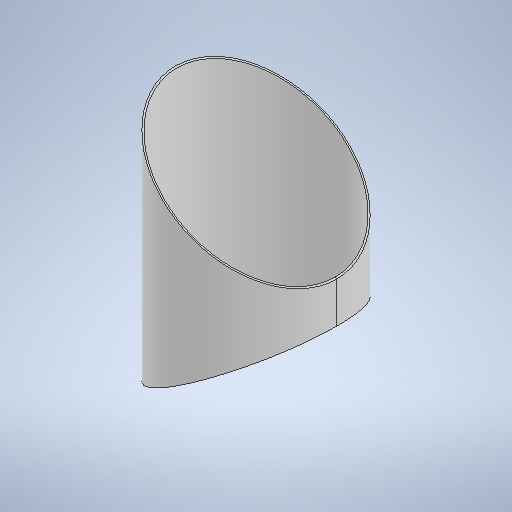
# Autodesk Inventor part: GBK-RK-0032 tube segmeng 2
Saved by Autodesk Inventor 2026.2 (Build 302298000, 298)
## iProperties
Created: 2026-09-14
Part Number: GBK-RK-0032 tube segmeng 2
Material: Generic
Document SubType Name: Sheet Metal
Designer: admin
Density: 1 g/cm^3
Flat Pattern Width: 101.018 cm
Flat Pattern Length: 50 cm
Flat Pattern Area: 5050.91 cm^2
Sheet Metal Rule: Default_mm
Sheet Metal Width: 1010,181 mm
Sheet Metal Length: 500,000 mm
Sheet Metal Area: 505090,589 mm^2
Appearance: Default
Author: admin
Autodesk Inventor part; units mm, degrees
ref_plane "YZ Plane" through (0, 0, 0) normal (1, 0, 0) x (0, 1, 0)
ref_plane "XZ Plane" through (0, 0, 0) normal (0, 1, 0) x (-1, 0, 0)
ref_plane "XY Plane" through (0, 0, 0) normal (0, 0, 1) x (1, 0, 0)
sketch "Sketch1" plane through (0, 0, 0) normal (0, 0, 1) x (1, 0, 0)
  line L0 (0, 0) -> (0, 204.8418)
  line L1 (159.5, 0) -> (162.5, 0)
  line L2 (162.5, 0) -> (162.5, 500)
  line L3 (162.5, 500) -> (159.5, 500)
  line L4 (159.5, 500) -> (159.5, 0)
  dimension "d0" = 3
  dimension "d1" = 500
  dimension "d2" = 325
  constraints: 10 end point, 2 parallel, 1 horizontal, 1 perpendicular, 1 point on line, 1 vertical
  measures "d0" distance of L3.end L2.end
  measures "d1" distance of L2.end L1.end
  measures "d2" diameter of L2 L0
revolve "Revolution1" add sketch "Sketch1" angle 359.9 about axis through (0, 0, 0) along (0, 1, 0)
sketch "Sketch2" plane through (0, 0, 0) normal (0, 0, 1) x (1, 0, 0)
  line L0 (162.5, 500) -> (-162.5, 500) projected
  line L1 (162.5, 0) -> (162.5, 500) projected
  line L2 (-162.5, 0) -> (-162.5, 500) projected
  line L3 (162.5, 0) -> (-162.5, 0) projected
  line L4 (-162.5, 0) -> (162.5, 208.8867)
  line L5 (-162.5, 500) -> (162.5, 291.1133)
  line L6 (-162.5, 250) -> (162.5, 250)
  point P0 (0, 0)
  point P1 (162.4998, 500)
  point P2 (162.4998, 0)
  dimension "d6" = 32.73
  constraints: 6 end point, 2 midpoint, 2 point on line, 1 other
  measures "d6" angle of L3 L4
extrude "Extrusion1" cut sketch "Sketch2" along normal through all both and the other way through all contours L1 L5 L0 | L4 L1 L3
equation "\"BendRadius\" = Thickness"
equation "\"BendReliefWidth\" = Thickness"
equation "\"BendReliefDepth\" = 0.5 * Thickness"
equation "\"CornerReliefSize\" = 4 * Thickness"
equation "\"MinimumRemnant\" = 2 * Thickness"
equation "\"TransitionRadius\" = BendRadius"
equation "\"JacobiRadiusSize\" = BendRadius"
equation "\"GapSize\" = Thickness"
equation "\"Thickness\" = 3"
body "Solid1"
